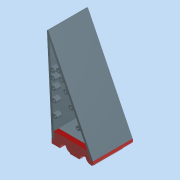
# Autodesk Inventor part: FingerEnclosure
Saved by Autodesk Inventor 2020.2 (Build 242310000, 310)
## iProperties
Created: 2020-03-10
Part Number: FingerEnclosure
Material: Generisch
Document SubType Name: Modeling
Designer: JochenAlt
Density: 1 g/cm^3
Appearance: Rot
Author: JochenAlt
Autodesk Inventor part; units mm, degrees
ref_plane "YZ Plane" through (0, 0, 0) normal (1, 0, 0) x (0, 1, 0)
ref_plane "XZ Plane" through (0, 0, 0) normal (0, 1, 0) x (-1, 0, 0)
ref_plane "XY Plane" through (0, 0, 0) normal (0, 0, 1) x (1, 0, 0)
sketch "MainConstruction" plane through (0, 0, 0) normal (0, 0, 1) x (1, 0, 0)
  line L0 (-44.4573, 0) -> (45.9096, 0) construction
  line L1 (0, -41.3) -> (0, 41.3) construction
  line L2 (-12, 16.3923) -> (12, 16.3923) construction
  line L3 (6, -16.3923) -> (6, -10.3923) construction
  line L4 (6, -10.3923) -> (11.1962, -13.3923) construction
  line L5 (8.1962, -18.5885) -> (11.1962, -13.3923) construction
  line L6 (0, -16.3923) -> (6, -16.3923) construction
  line L7 (-6, -10.3923) -> (-6, -16.3923) construction
  line L8 (-6, -10.3923) -> (-11.1962, -13.3923) construction
  line L9 (0, 16.3923) -> (0, 0) construction
  line L10 (0, 0) -> (0, -16.3923) construction
  line L11 (-12, 14.3923) -> (12, 14.3923) construction
  line L12 (-12, 16.3923) -> (-12, 14.3923) construction
  line L13 (-12, 27) -> (12, 27) construction
  line L14 (-29.3827, -3.1077) -> (-17.3827, -23.8923) construction
  line L15 (0, 16.3923) -> (0, 27) construction
  line L16 (-23.3827, -13.5) -> (-14.1962, -8.1962) construction
  arc A0 (-2.6277, -14.0839) -> (-3.3698, -6.14) centre (-6, -10.3923) ccw construction
  arc A1 (3.3698, -6.14) -> (2.6277, -14.0839) centre (6, -10.3923) ccw construction
  line L17 (-27.2176, -1.8577) -> (-31.5477, -4.3577) construction
  line L18 (-15.2176, -22.6423) -> (-19.5477, -25.1423) construction
  line L19 (19.5477, -25.1423) -> (15.2176, -22.6423) construction
  circle A2 centre (0, 0) radius 22 construction
  line L20 (12, 14.3923) -> (12, 16.3923) construction
  line L21 (23.3827, -13.5) -> (14.1962, -8.1962) construction
  line L22 (20.1962, 2.1962) -> (14.1962, -8.1962) construction
  line L23 (11.1962, -13.3923) -> (14.1962, -8.1962) construction
  line L24 (-6, -16.3923) -> (0, -16.3923) construction
  line L25 (8.1962, -18.5885) -> (15.2176, -22.6423) construction
  line L26 (-15.2176, -22.6423) -> (-8.1962, -18.5885) construction
  line L27 (-12, 29.5) -> (-12, 24.5) construction
  line L28 (12, 29.5) -> (12, 24.5) construction
  line L29 (12, 24.5) -> (12, 16.3923) construction
  line L30 (-12, 24.5) -> (-12, 16.3923) construction
  line L31 (-11.1962, -13.3923) -> (-8.1962, -18.5885) construction
  line L32 (-11.1962, -13.3923) -> (-20.1962, 2.1962) construction
  line L33 (27.2176, -1.8577) -> (31.5477, -4.3577) construction
  line L34 (17.3827, -23.8923) -> (29.3827, -3.1077) construction
  line L35 (27.2176, -1.8577) -> (21.9687, 1.1728) construction
  line L36 (-27.2176, -1.8577) -> (-21.9687, 1.1728) construction
  line L37 (20.1962, 2.1962) -> (21.9687, 1.1728) construction
  line L38 (-21.9687, 1.1728) -> (-20.1962, 2.1962) construction
  line L39 (0, -16.3923) -> (0, -24.5) construction
  line L40 (0, -24.5) -> (0, -29.5) construction
  line L41 (0, -27) -> (24, -27) construction
  line L42 (18.4641, 3.1962) -> (6.4641, -17.5885) construction
  line L43 (-18.4641, 3.1962) -> (-6.4641, -17.5885) construction
  line L44 (-20.1962, 2.1962) -> (-18.4641, 3.1962) construction
  line L45 (20.1962, 2.1962) -> (18.4641, 3.1962) construction
  line L46 (3.3698, -6.14) -> (18.4641, 3.1962) construction
  line L47 (-18.4641, 3.1962) -> (-3.3698, -6.14) construction
  circle A3 centre (30.5, 27) radius 2.5 construction
  line L48 (12, 14.3923) -> (16.25, 14.3923) construction
  line L49 (16.25, 14.3923) -> (31.8962, 24.9262) construction
  line L50 (29.1038, 29.0738) -> (10.2677, 16.3923) construction
  line L51 (12, 16.3923) -> (10.2677, 16.3923) construction
  line L52 (8.1962, -18.5885) -> (6.4641, -17.5885) construction
  line L53 (6.4641, -17.5885) -> (2.6277, -14.0839) construction
  line L54 (-8.1962, -18.5885) -> (-6.4641, -17.5885) construction
  line L55 (-6.4641, -17.5885) -> (-2.6277, -14.0839) construction
  line L56 (4.7294, -16.5869) -> (6.4641, -17.5885) construction
sketch "Main" plane through (0, 0, 0) normal (0, 0, 1) x (1, 0, 0)
  line L0 (-20, 3) -> (-22.8717, 57.562)
  line L1 (-23, 60) -> (-21.9236, 57.8088) construction
  line L2 (5, 3) -> (-20, 3)
  line L3 (-13.0482, 36.6791) -> (-12.4971, 35.5572) construction
  line L4 (-19.213, 13.7322) -> (-18.7534, 5)
  line L5 (-19.598, 21.0479) -> (-19.6335, 21.7211) construction
  line L6 (-19.9698, 28.1122) -> (-19.7648, 24.2176)
  line L7 (-6.7583, 23.8747) -> (-3.6016, 17.4486)
  line L8 (-10.0113, 30.4969) -> (-7.8606, 26.1186)
  line L9 (-21.3054, 53.4884) -> (-15.4967, 41.6635)
  line L10 (-12.4971, 35.5572) -> (-11.1136, 32.7408)
  line L11 (-21.3054, 53.4884) -> (-20.5856, 39.8121)
  line L12 (-20.2389, 33.2252) -> (-20.1012, 30.6088)
  line L13 (-3.0505, 16.3266) -> (-2.4994, 15.2047) construction
  line L14 (-3.6016, 17.4486) -> (-3.0505, 16.3266) construction
  line L15 (-2.4994, 15.2047) -> (2.5135, 5) construction
  line L16 (-19.3444, 16.2287) -> (-19.598, 21.0479) construction
  line L17 (-19.2787, 14.9804) -> (-19.3444, 16.2287) construction
  line L18 (-19.213, 13.7322) -> (-19.2787, 14.9804) construction
  line L19 (-7.8606, 26.1186) -> (-7.3094, 24.9966) construction
  line L20 (-7.3094, 24.9966) -> (-6.7583, 23.8747) construction
  line L21 (-6.7583, 23.8747) -> (-3.6016, 17.4486) construction
  line L22 (-19.598, 21.0479) -> (-19.6992, 22.9694) construction
  line L23 (-20.1012, 30.6088) -> (-20.2389, 33.2252) construction
  line L24 (-20.0355, 29.3605) -> (-20.1012, 30.6088) construction
  line L25 (-19.9698, 28.1122) -> (-20.0355, 29.3605) construction
  line L26 (-11.1136, 32.7408) -> (-10.5625, 31.6188) construction
  line L27 (-10.5625, 31.6188) -> (-10.0113, 30.4969) construction
  line L28 (-10.0113, 30.4969) -> (-7.8606, 26.1186) construction
  line L29 (-20.3703, 35.7217) -> (-20.3046, 34.4734) construction
  line L30 (-13.5993, 37.801) -> (-13.0482, 36.6791) construction
  line L31 (-12.4971, 35.5572) -> (-11.1136, 32.7408) construction
  line L32 (-20.2389, 33.2252) -> (-20.3046, 34.4734) construction
  line L33 (-18.7534, 5) -> (-19.213, 13.7322) construction
  line L34 (-2.4994, 15.2047) -> (2.5135, 5)
  line L35 (-18.7534, 5) -> (2.5135, 5)
  arc A0 (-21.9236, 57.8088) -> (-22.8717, 57.562) centre (-22.3724, 57.5883) ccw
  line L36 (-18.7534, 5) -> (-18.6481, 3)
  line L37 (2.5135, 5) -> (3.4959, 3)
  circle A1 centre (-12, 0) radius 1.05
  arc A2 (-14.9041, -0.7524) -> (-9, 0) centre (-12, 0) ccw
  circle A3 centre (0, 0) radius 1.05
  arc A4 (-3, 0) -> (3, 0) centre (0, 0) ccw
  line L38 (-9, 0) -> (-3, 0)
  line L39 (3, 0) -> (3.1313, 0)
  arc A5 (3.1313, 0) -> (5, 3) centre (3.1313, 2.082) ccw
  line L40 (-18.7585, 7) -> (1.4196, 7)
  line L41 (-18.6533, 5) -> (-18.7585, 7)
  line L42 (1.4196, 7) -> (2.402, 5)
  line L43 (-18.6585, 5.1) -> (2.3529, 5.1)
  arc A6 (3, 0) -> (-3, 0) centre (0, 0) ccw
  line L44 (2.1213, 2.1213) -> (4.0359, 0.2068)
  arc A7 (-9, 0) -> (-14.9041, -0.7524) centre (-12, 0) ccw
  line L45 (2.402, 5) -> (3.3845, 3)
  line L46 (-18.6533, 5) -> (-18.548, 3)
  line L47 (-20, 3) -> (-20, 0)
  line L48 (-21.9236, 57.8088) -> (5, 3)
  line L49 (-22.8717, 57.562) -> (-23, 60) construction
  line L50 (-23, 60) -> (-23, 0) construction
  line L51 (0, -47.4) -> (0, 77.9) construction
  line L52 (-44.4573, 0) -> (45.9096, 0) construction
  line L53 (3, 0) -> (-23, 0) construction
  arc A8 (-14.9041, -0.7524) -> (-14.9041, -0.7524) centre (-12, 0) ccw
  line L54 (-15, 0) -> (-20, 0)
  line L55 (-15.2356, 0) -> (-14.7816, 1.1238)
  line L56 (-9.1468, 0.9271) -> (-8.8456, 0)
  line L57 (-8.8456, 0) -> (-9.1468, -0.9271)
  line L58 (-15.2356, 0) -> (-14.7816, -1.1238)
  line L59 (-2.7615, 1.1722) -> (-3.2591, 0)
  line L60 (-2.7615, -1.1722) -> (-3.2591, 0)
  line L61 (-20.3703, 35.7217) -> (-19.1221, 35.7874)
  arc A9 (-18.9907, 33.2909) -> (-19.1221, 35.7874) centre (-19.0564, 34.5391) ccw
  line L62 (-18.9907, 33.2909) -> (-20.2389, 33.2252)
  line L63 (-13.5993, 37.801) -> (-14.7213, 37.2499)
  arc A10 (-14.7213, 37.2499) -> (-13.619, 35.006) centre (-14.1702, 36.128) ccw
  line L64 (-13.619, 35.006) -> (-12.4971, 35.5572)
  line L65 (-11.1136, 32.7408) -> (-12.2355, 32.1897)
  arc A11 (-12.2355, 32.1897) -> (-11.1333, 29.9458) centre (-11.6844, 31.0677) ccw
  line L66 (-11.1333, 29.9458) -> (-10.0113, 30.4969)
  line L67 (-20.1012, 30.6088) -> (-18.853, 30.6745)
  arc A12 (-18.7216, 28.1779) -> (-18.853, 30.6745) centre (-18.7873, 29.4262) ccw
  line L68 (-18.7216, 28.1779) -> (-19.9698, 28.1122)
  line L69 (-7.8606, 26.1186) -> (-8.9825, 25.5674)
  arc A13 (-8.9825, 25.5674) -> (-7.8803, 23.3235) centre (-8.4314, 24.4455) ccw
  line L70 (-7.8803, 23.3235) -> (-6.7583, 23.8747)
  line L71 (-3.6016, 17.4486) -> (-4.7236, 16.8974)
  arc A14 (-4.7236, 16.8974) -> (-3.6213, 14.6535) centre (-4.1724, 15.7755) ccw
  line L72 (-3.6213, 14.6535) -> (-2.4994, 15.2047)
  line L73 (-19.3444, 16.2287) -> (-18.0961, 16.2944)
  arc A15 (-17.9647, 13.7978) -> (-18.0961, 16.2944) centre (-18.0304, 15.0461) ccw
  line L74 (-17.9647, 13.7978) -> (-19.213, 13.7322)
  arc A16 (-13.619, 35.006) -> (-14.7213, 37.2499) centre (-14.1702, 36.128) ccw construction
  circle A17 centre (-14.1702, 36.128) radius 0.5
  circle A18 centre (-19.0564, 34.5391) radius 0.5
  circle A19 centre (-18.7873, 29.4262) radius 0.5
  arc A20 (-19.1221, 35.7874) -> (-17.8066, 34.5618) centre (-19.0564, 34.5391) ccw construction
  arc A21 (-18.853, 30.6745) -> (-18.7216, 28.1779) centre (-18.7873, 29.4262) ccw construction
  circle A22 centre (-11.6844, 31.0677) radius 0.5
  circle A23 centre (-8.4314, 24.4455) radius 0.5
  arc A24 (-7.8803, 23.3235) -> (-8.9825, 25.5674) centre (-8.4314, 24.4455) ccw construction
  circle A25 centre (-18.0304, 15.0461) radius 0.5
  arc A26 (-18.0961, 16.2944) -> (-17.9647, 13.7978) centre (-18.0304, 15.0461) ccw construction
  circle A27 centre (-4.1724, 15.7755) radius 0.5
  arc A28 (-3.6213, 14.6535) -> (-4.7236, 16.8974) centre (-4.1724, 15.7755) ccw construction
  line L75 (-19.0564, 34.5391) -> (-14.1702, 36.128) construction
  line L76 (-18.7873, 29.4262) -> (-11.6844, 31.0677) construction
  line L77 (-18.0304, 15.0461) -> (-4.1724, 15.7755) construction
  circle A29 centre (-19.2716, 38.6295) radius 0.5
  arc A30 (-20.5199, 38.5638) -> (-19.2059, 37.3812) centre (-19.2716, 38.6295) ccw construction
  line L78 (-19.3373, 39.8778) -> (-20.5856, 39.8121)
  line L79 (-20.4542, 37.3155) -> (-19.2059, 37.3812)
  arc A31 (-19.3373, 39.8778) -> (-20.5199, 38.5638) centre (-19.2716, 38.6295) ccw construction
  arc A32 (-19.2059, 37.3812) -> (-19.3373, 39.8778) centre (-19.2716, 38.6295) ccw
  line L80 (-20.4542, 37.3155) -> (-20.3703, 35.7217)
  line L81 (-20.5856, 39.8121) -> (-20.4542, 37.3155)
  circle A33 centre (-16.0675, 39.9904) radius 0.5
  arc A34 (-16.6186, 41.1123) -> (-15.5164, 38.8685) centre (-16.0675, 39.9904) ccw
  line L82 (-16.6186, 41.1123) -> (-15.4967, 41.6635)
  line L83 (-15.5164, 38.8685) -> (-14.3944, 39.4196)
  arc A35 (-14.9455, 40.5415) -> (-16.6186, 41.1123) centre (-16.0675, 39.9904) ccw construction
  arc A36 (-15.5164, 38.8685) -> (-14.9455, 40.5415) centre (-16.0675, 39.9904) ccw construction
  line L84 (-14.3944, 39.4196) -> (-13.5993, 37.801)
  line L85 (-15.4967, 41.6635) -> (-14.3944, 39.4196) construction
  line L86 (-19.2716, 38.6295) -> (-16.0675, 39.9904) construction
  circle A37 centre (-18.4509, 23.0351) radius 0.5
  arc A38 (-19.6992, 22.9694) -> (-18.3852, 21.7868) centre (-18.4509, 23.0351) ccw construction
  line L87 (-18.5166, 24.2833) -> (-19.7648, 24.2176)
  line L88 (-18.3852, 21.7868) -> (-19.6335, 21.7211)
  arc A39 (-18.5166, 24.2833) -> (-19.6992, 22.9694) centre (-18.4509, 23.0351) ccw construction
  arc A40 (-18.3852, 21.7868) -> (-18.5166, 24.2833) centre (-18.4509, 23.0351) ccw
  line L89 (-19.6335, 21.7211) -> (-19.3444, 16.2287)
  line L90 (-18.4509, 23.0351) -> (-8.4314, 24.4455) construction
  line L91 (-19.7648, 24.2176) -> (-19.6992, 22.9694) construction
  line L92 (-18.7585, 7) -> (-18.8584, 6.9947)
  line L93 (1.4196, 7) -> (1.531, 7)
  arc A41 (-11.1333, 29.9458) -> (-12.2355, 32.1897) centre (-11.6844, 31.0677) ccw construction
  point P0 (-20.0699, 4.3273)
  point P1 (-18.588, 1.8575)
  point P2 (0, 3)
  point P3 (-12, 3)
  point P4 (11.0172, 9.525)
  point P5 (3.5032, 0.0324)
  point P6 (-16.5, 3)
  point P7 (-3.2591, 0)
  point P8 (-14.9041, -0.7524)
  point P9 (-19.6992, 22.9694)
  dimension "d29" = 1.35
  dimension "d30" = 1.35
  dimension "d45" = 0.5
  dimension "d46" = 2
  dimension "d112" = 2.1
  dimension "d114" = 12
  dimension "d124" = 2
  dimension "d127" = 0.1
  dimension "d128" = 0.1
  dimension "d129" = 0.1
  dimension "d133" = 25
  dimension "d138" = 60
  dimension "d141" = 10
  dimension "d142" = 8
  dimension "d143" = 6.4
  dimension "d144" = 5.12
  dimension "d145" = 8
  dimension "d147" = 68
  dimension "d148" = 135
  dimension "d149" = 72
  dimension "d150" = 67
  dimension "d151" = 3
  dimension "d152" = 3
  dimension "d154" = 3
  dimension "d155" = 1
  dimension "d156" = 1.25
  dimension "d163" = 4.096
  dimension "d164" = 70
  dimension "d165" = 5
  dimension "d166" = 5
  dimension "d167" = 5
  dimension "d168" = 5
  constraints: 186 end point, 174 collinear, 82 point on circle, 65 tangent, 42 centre point, 33 point on line, 30 perpendicular, 22 equal radius, 19 coincident, 7 horizontal, 6 parallel, 2 midpoint, 1 vertical, 9 other
  measures "d29" distance between parallel lines of L0 L11
  measures "d30" distance between parallel lines of L1 L9
  measures "d45" radius of A0
  measures "d46" distance between parallel lines of L2 L35
  measures "d112" diameter of A1
  measures "d114" distance of A3.centre A1.centre
  measures "d124" distance between parallel lines of L40 L35
  measures "d127" distance between parallel lines of L41 L4
  measures "d128" distance between parallel lines of L34 L42
  measures "d129" distance between parallel lines of L43 L35
  measures "d133" distance of L2.start L0.start
  measures "d138" distance of L1.start L50.end
  measures "d141" distance of L17.start L41.start
  measures "d142" distance of L17.start L22.end
  measures "d143" distance of L22.end L24.start
  measures "d144" distance of L32.end L24.start
  measures "d145" distance from line of A7.centre L47
  measures "d147" angle of L54 L55
  measures "d148" angle of L52 L44
  measures "d149" angle of L38 L56
  measures "d150" angle of L38 L59
  measures "d151" radius of A2
  measures "d152" distance between parallel lines of L2 L53
  measures "d154" distance of L47.end L50.end
  measures "d155" diameter of A17
  measures "d156" radius of A10
  measures "d163" distance of L32.end A30.start
  measures "d164" angle of L86 L11
  measures "d165" angle of L90 L76
  measures "d166" angle of L77 L90
  measures "d167" angle of L75 L86
  measures "d168" angle of L76 L75
extrude "Extrusion1" add sketch "Main" along normal mid plane 18 contours L0 A0 L48 L2 L37 L34 L72 A14 L71 L7 L70 A13 L69 L8 L66 A11 L65 L10 L64 A10 L63 L84 L83 A34 L82 L9 L11 L81 L80 L61 A9 L62 L12 L67 A12 L68 L6 L87 A40 L88 L89 L73 A15 L74 L4 L36 | L36 L35 L46 L2 | L46 L35 L45 L2 | L4 L92 L41 L35 | L41 L43 L42 L35 | L2 L45 L35 L37 | L42 L93 L34 L35 | L41 L40 L42 L43 | L81 L78 A32 L79
extrude "Extrusion16" add sketch "Main" along normal mid plane 24 contours L0 A0 L48 L2 L37 L34 L72 A14 L71 L7 L70 A13 L69 L8 L66 A11 L65 L10 L64 A10 L63 L84 L83 A34 L82 L9 L11 L81 L80 L61 A9 L62 L12 L67 A12 L68 L6 L87 A40 L88 L89 L73 A15 L74 L4 L36 | L81 L78 A32 L79
sketch "Skizze5" plane through (0, 0, 0) normal (0, 0, 1) x (1, 0, 0)
  line L0 (2.5135, 5) -> (-21.3054, 53.4884)
  line L1 (-18.7534, 5) -> (2.5135, 5)
  line L2 (2.5135, 5) -> (-18.7534, 5)
  line L3 (-20.3703, 35.7217) -> (-21.3054, 53.4884) construction
  line L4 (-18.7534, 5) -> (-21.3054, 53.4884)
  line L5 (-18.6481, 3) -> (-19.213, 13.7322) projected
  line L6 (-18.8587, 7) -> (1.531, 7)
  line L7 (1.4196, 7) -> (-18.7585, 7) projected
  point P0 (0, 0)
  constraints: 10 end point, 3 collinear, 3 point on line, 1 coincident, 1 horizontal
extrude "Extrusion21" cut sketch "Skizze5" along normal mid plane 18 contours L6 L4 L0
extrude "Extrusion17" add sketch "Main" along normal mid plane 17 separate body contours L2 A7 L55 L54 L47 | L55 A7 L54 | L54 A7 A2 L58 | A5 L44 A6 L2 | L2 A6 L59 L38 L56 A7 | A7 A2 | A5 L39 A6 L44 | A6 A4 | L56 L38 A7 | A2 L38 L57 | A6 L38 L59 | A4 L60 L38
extrude "Extrusion18" add sketch "Main" along normal mid plane 24 contours L2 A7 L55 L54 L47 | L46 L35 L45 L2 | L55 A7 L54 | A5 L44 A6 L2 | L2 A6 L59 L38 L56 A7 | L41 L43 L42 L35 | L41 L40 L42 L43 bodies 2
extrude "Extrusion19" cut sketch "Main" along normal mid plane 20.25 contours L36 L35 L46 L2 | L46 L35 L45 L2 | L41 L43 L42 L35 | L2 L45 L35 L37 bodies 2
extrude "Extrusion20" cut sketch "Main" along normal mid plane 18 contours L41 L43 L42 L35 | L41 L40 L42 L43 bodies 2
equation "\"d30\" = d29"
equation "\"d5\" = d20"
equation "\"roundness_small\" = 3"
equation "\"roundness_tiny\" = 0.5"
equation "\"wall_thickness\" = 3"
equation "\"medium_arm_width\" = 51"
equation "\"big_arm_width\" = 56"
equation "\"bevel_angle\" = 20deg"
equation "\"medium_arm_radius\" = 35"
equation "\"big_arm_radius\" = 48"
equation "\"medium_arm_circle_centre\" = 11"
equation "\"big_arm_circle_centre\" = 25"
equation "\"thickness\" = 3"
equation "\"tight_fit\" = 0.2"
equation "\"press_fit\" = 0.1"
equation "\"m2_screw_hole_diameter\" = 2.2"
equation "\"m2_hex_width\" = 4.2"
equation "\"m2_washer_diameter\" = 5.2"
equation "\"m2_allen_screw_width\" = 4"
equation "\"m2_allen_screw_height\" = 2"
equation "\"m2_washer_height\" = 0.3"
equation "\"d20\" = 1"
